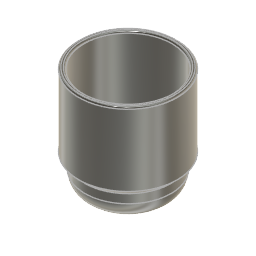
basic_self_watering_potjie (Autodesk Fusion 360 design; units mm, degrees)
Autodesk Fusion 360 part; units mm, degrees
sketch "simple_potjie_base" plane through (0, 0, 0) normal (0, 0, 1) x (1, 0, 0)
  circle A0 centre (0, 0) radius 25
  circle A1 centre (0, 0) radius 28
  circle A2 centre (0, 0) radius 22
  line L0 (0, 0) -> (-7, 0)
  line L1 (0, 0) -> (7, 0)
  circle A3 centre (7, 0) radius 4
  circle A4 centre (-7, 0) radius 4
  dimension "d4" = 50
  dimension "d5" = 56
  dimension "d36" = 44
  dimension "d46" = 7
  dimension "d47" = 7
  dimension "d48" = 8
  dimension "d49" = 8
  constraint coincident A0.centre A1.centre
  constraint concentric A1 A2
  constraint horizontal L0
  constraint parallel L0 L1
  constraint coincident L1.end A3.centre
  constraint coincident L0.end A4.centre
  measures "d4" diameter of A0
  measures "d5" diameter of A1
  measures "d36" diameter of A2
  measures "d46" distance of A0.centre L0.end
  measures "d47" distance of A0.centre L1.end
  measures "d48" diameter of A3
  measures "d49" diameter of A4
extrude "Extrude1" add sketch "simple_potjie_base" along normal blind 3 contours A0 | A2 | A3 | A4 makes body 1
extrude "Extrude2" add sketch "simple_potjie_base" along normal blind 60 and the other way blind -15 separate body contours A1 makes body 2
chamfer "Chamfer2" distance 3 angle 45 1 edges at (-23.3082, -9.0404, 3) on bodies 1
extrude "Extrude4" add sketch "simple_potjie_base" along normal blind 18 contours A0 bodies 1 2
chamfer "Chamfer4" distance 3 angle 45 1 edges at (-23.3082, 9.0404, 18) on bodies 1
fillet "Fillet5" radius 7 1 edges at (-20.5112, 7.9555, 3) on bodies 1
fillet "Fillet6" radius 10 1 edges at (-23.3082, -9.0404, 0) on bodies 1
extrude "Extrude5" cut sketch "simple_potjie_base" along normal blind 3 contours A3 | A4 bodies 1
fillet "Fillet7" radius 1 2 edges at (-26.1052, -10.1252, 60) (-23.3082, 9.0404, 60) on bodies 1 2
move_face "OffsetFaces1" offset -0.5 1 faces at (-24.8758, -2.4892, 11.6667) on bodies 1
chamfer "Chamfer5" distance 3.5 angle 45 1 edges at (-26.1052, -10.1252, 15) on bodies 1
equation "wall_thinkness = 3 mm" comment "Thickness of the walls of the entire print."
equation "pot_height = 60 mm" comment "Total height of the pot. Including the narrowing insert part."
equation "pot_inner_diameter = 50 mm" comment "Inner diameter of the upper part of the pot."
equation "d4 = pot_inner_diameter"
equation "d5 = pot_inner_diameter + ( 2 * wall_thinkness )"
equation "d6 = wall_thinkness"
equation "d8 = pot_height"
equation "pot_bottom_fillet = 10 mm" comment "Fillet/Rounding of the bottom of the pot. Inner fillet calculated automatically."
equation "pot_finger_cutout_num = 2" comment "Number of finger cutouts around the upper brim."
equation "pot_finger_cutout_width = 20 mm" comment "Width of the finger cutout."
equation "pot_finger_cutout_height = 7 mm" comment "Height of the finger cutout."
equation "d31 = wall_thinkness"
equation "d33 = -pot_bottom_insert_height"
equation "pot_bottom_insert_height = 15 mm" comment "The height of the bottom narrower portion that will fit into the lower pot."
equation "d36 = pot_inner_diameter - ( 2 * wall_thinkness )"
equation "d37 = pot_bottom_insert_height + wall_thinkness"
equation "d39 = wall_thinkness"
equation "d41 = pot_bottom_fillet - wall_thinkness"
equation "d43 = pot_bottom_fillet"
equation "wick_holes_distance_apart = 6 mm" comment "Distance between the holes for the wick to go through."
equation "wick_hole_diameter = 8 mm" comment "Diameter of the holes for the wick to go through."
equation "d46 = wick_holes_distance_apart / 2 + wick_hole_diameter / 2"
equation "d47 = wick_holes_distance_apart / 2 + wick_hole_diameter / 2"
equation "d48 = wick_hole_diameter"
equation "d49 = wick_hole_diameter"
equation "d50 = wall_thinkness"
named bodies: "simple_potjie"
